Autodesk Inventor part; units mm, degrees
(part 3 of 3)
  spline S531 degree 2 poles (91.9053, 44.1267) (92.1175, 44.1267) (92.457, 44.0701) (92.5051, 44.0362) knots 0 0 0 1 2 2 2
  line L562 (92.5051, 44.0362) -> (92.5051, 43.3289)
  spline S532 degree 2 poles (92.5051, 43.3289) (92.4372, 43.3826) (92.1826, 43.4618) (92.0751, 43.4618) knots 0 0 0 1 2 2 2
  spline S533 degree 2 poles (92.0751, 43.4618) (91.8091, 43.4618) (91.5347, 43.21) (91.5347, 42.9808) knots 0 0 0 1 2 2 2
  spline S534 degree 2 poles (91.5347, 42.9808) (91.5347, 42.7545) (91.8035, 42.5055) (92.0411, 42.5055) knots 0 0 0 1 2 2 2
  spline S535 degree 2 poles (92.0411, 42.5055) (92.2929, 42.5055) (92.5051, 42.6244) knots 0 0 0 1 1 1
  line L563 (92.5051, 42.6244) -> (92.5051, 41.9566)
  spline S536 degree 2 poles (93.6482, 42.7262) (93.6708, 42.5847) (93.9481, 42.4263) (94.1744, 42.4263) knots 0 0 0 1 2 2 2
  spline S537 degree 2 poles (94.1744, 42.4263) (94.4913, 42.4263) (94.7742, 42.548) knots 0 0 0 1 1 1
  line L564 (94.7742, 42.548) -> (94.7742, 41.9736)
  spline S538 degree 2 poles (94.7742, 41.9736) (94.446, 41.8406) (93.9735, 41.8406) knots 0 0 0 1 1 1
  spline S539 degree 2 poles (93.9735, 41.8406) (93.4048, 41.8406) (92.7711, 42.4235) (92.7711, 42.9356) knots 0 0 0 1 2 2 2
  spline S540 degree 2 poles (92.7711, 42.9356) (92.7711, 43.2864) (93.0484, 43.8212) (93.5944, 44.1267) (93.9254, 44.1267) knots 0 0 0 1 2 3 3 3
  spline S541 degree 2 poles (93.9254, 44.1267) (94.2621, 44.1267) (94.7431, 43.8636) (94.9921, 43.3854) (94.9921, 43.0657) knots 0 0 0 1 2 3 3 3
  line L565 (94.9921, 43.0657) -> (94.9921, 42.7262)
  line L566 (94.9921, 42.7262) -> (93.6482, 42.7262)
  spline S542 degree 2 poles (94.1914, 43.2015) (94.1914, 43.5778) (93.9226, 43.5778) knots 0 0 0 1 1 1
  spline S543 degree 2 poles (93.9226, 43.5778) (93.8094, 43.5778) (93.6567, 43.3713) (93.6425, 43.2015) knots 0 0 0 1 2 2 2
  line L567 (93.6425, 43.2015) -> (94.1914, 43.2015)
  line L568 (96.718, 41.8944) -> (96.718, 43.0827)
  spline S544 degree 2 poles (96.718, 43.0827) (96.718, 43.2864) (96.5963, 43.4618) (96.4605, 43.4618) knots 0 0 0 1 2 2 2
  spline S545 degree 2 poles (96.4605, 43.4618) (96.3445, 43.4618) (96.2115, 43.2779) (96.2115, 43.1365) knots 0 0 0 1 2 2 2
  line L569 (96.2115, 43.1365) -> (96.2115, 41.8944)
  line L570 (96.2115, 41.8944) -> (95.3061, 41.8944)
  line L571 (95.3061, 41.8944) -> (95.3061, 44.073)
  line L572 (95.3061, 44.073) -> (96.2115, 44.073)
  line L573 (96.2115, 44.073) -> (96.2115, 43.7334)
  line L574 (96.2115, 43.7334) -> (96.22, 43.7334)
  spline S546 degree 2 poles (96.22, 43.7334) (96.3275, 43.9202) (96.6953, 44.1267) (96.9104, 44.1267) knots 0 0 0 1 2 2 2
  spline S547 degree 2 poles (96.9104, 44.1267) (97.6234, 44.1267) (97.6234, 43.2242) knots 0 0 0 1 1 1
  line L575 (97.6234, 43.2242) -> (97.6234, 41.8944)
  line L576 (97.6234, 41.8944) -> (96.718, 41.8944)
  line L577 (99.0578, 42.5225) -> (99.9547, 42.5225)
  line L578 (99.9547, 42.5225) -> (99.9547, 41.8944)
  line L579 (99.9547, 41.8944) -> (97.8695, 41.8944)
  line L580 (97.8695, 41.8944) -> (97.8695, 42.3131)
  line L581 (97.8695, 42.3131) -> (98.8484, 43.4449)
  line L582 (98.8484, 43.4449) -> (97.96, 43.4449)
  line L583 (97.96, 43.4449) -> (97.96, 44.073)
  line L584 (97.96, 44.073) -> (99.9349, 44.073)
  line L585 (99.9349, 44.073) -> (99.9349, 43.558)
  line L586 (99.9349, 43.558) -> (99.0578, 42.5225)
  spline S548 degree 2 poles (102.6737, 43.0233) (102.6737, 42.4716) (102.0088, 41.8406) (101.4118, 41.8406) knots 0 0 0 1 2 2 2
  spline S549 degree 2 poles (101.4118, 41.8406) (100.8177, 41.8406) (100.1556, 42.4546) (100.1556, 42.9978) knots 0 0 0 1 2 2 2
  spline S550 degree 2 poles (100.1556, 42.9978) (100.1556, 43.343) (100.4668, 43.8551) (101.0412, 44.1267) (101.4146, 44.1267) knots 0 0 0 1 2 3 3 3
  spline S551 degree 2 poles (101.4146, 44.1267) (101.8023, 44.1267) (102.3709, 43.841) (102.6737, 43.3345) (102.6737, 43.0233) knots 0 0 0 1 2 3 3 3
  spline S552 degree 2 poles (101.7542, 43.0176) (101.7542, 43.4618) (101.4146, 43.4618) knots 0 0 0 1 1 1
  spline S553 degree 2 poles (101.4146, 43.4618) (101.0751, 43.4618) (101.0751, 42.9978) knots 0 0 0 1 1 1
  spline S554 degree 2 poles (101.0751, 42.9978) (101.0751, 42.5055) (101.4203, 42.5055) knots 0 0 0 1 1 1
  spline S555 degree 2 poles (101.4203, 42.5055) (101.7542, 42.5055) (101.7542, 43.0176) knots 0 0 0 1 1 1
  line L587 (105.2257, 44.2257) -> (105.2257, 43.6769)
  line L588 (105.2257, 43.6769) -> (106.1311, 43.6769)
  line L589 (106.1311, 43.6769) -> (106.1311, 42.9582)
  line L590 (106.1311, 42.9582) -> (105.2257, 42.9582)
  line L591 (105.2257, 42.9582) -> (105.2257, 41.8944)
  line L592 (105.2257, 41.8944) -> (104.3062, 41.8944)
  line L593 (104.3062, 41.8944) -> (104.3062, 44.9444)
  line L594 (104.3062, 44.9444) -> (106.2188, 44.9444)
  line L595 (106.2188, 44.9444) -> (106.2188, 44.2257)
  line L596 (106.2188, 44.2257) -> (105.2257, 44.2257)
  line L597 (107.7891, 41.8944) -> (107.7891, 42.2254)
  line L598 (107.7891, 42.2254) -> (107.7806, 42.2254)
  spline S556 degree 2 poles (107.7806, 42.2254) (107.5627, 41.8406) (107.1157, 41.8406) knots 0 0 0 1 1 1
  spline S557 degree 2 poles (107.1157, 41.8406) (106.8073, 41.8406) (106.4593, 42.2056) (106.4593, 42.514) knots 0 0 0 1 2 2 2
  spline S558 degree 2 poles (106.4593, 42.514) (106.4593, 43.1563) (107.2487, 43.2581) knots 0 0 0 1 1 1
  line L599 (107.2487, 43.2581) -> (107.7891, 43.3289)
  spline S559 degree 2 poles (107.7891, 43.3289) (107.7891, 43.4364) (107.5967, 43.5722) (107.4354, 43.5722) knots 0 0 0 1 2 2 2
  spline S560 degree 2 poles (107.4354, 43.5722) (107.0704, 43.5722) (106.663, 43.3628) knots 0 0 0 1 1 1
  line L600 (106.663, 43.3628) -> (106.663, 43.9513)
  spline S561 degree 2 poles (106.663, 43.9513) (106.8384, 44.0277) (107.3732, 44.1267) (107.5627, 44.1267) knots 0 0 0 1 2 2 2
  spline S562 degree 2 poles (107.5627, 44.1267) (108.1173, 44.1267) (108.6181, 43.6514) (108.6181, 43.0968) knots 0 0 0 1 2 2 2
  line L601 (108.6181, 43.0968) -> (108.6181, 41.8944)
  line L602 (108.6181, 41.8944) -> (107.7891, 41.8944)
  spline S563 degree 2 poles (107.2515, 42.6357) (107.2515, 42.548) (107.3647, 42.432) (107.4694, 42.432) knots 0 0 0 1 2 2 2
  spline S564 degree 2 poles (107.4694, 42.432) (107.6108, 42.432) (107.7891, 42.6442) (107.7891, 42.8111) knots 0 0 0 1 2 2 2
  line L603 (107.7891, 42.8111) -> (107.7891, 42.8931)
  line L604 (107.7891, 42.8931) -> (107.4807, 42.8507)
  spline S565 degree 2 poles (107.4807, 42.8507) (107.2515, 42.8111) (107.2515, 42.6357) knots 0 0 0 1 1 1
  spline S566 degree 2 poles (111.4813, 43.0488) (111.4813, 42.6923) (111.2465, 42.1405) (110.8108, 41.8406) (110.5363, 41.8406) knots 0 0 0 1 2 3 3 3
  spline S567 degree 2 poles (110.5363, 41.8406) (110.327, 41.8406) (110.0271, 41.9962) (109.9394, 42.1207) knots 0 0 0 1 2 2 2
  line L605 (109.9394, 42.1207) -> (109.9309, 42.1207)
  line L606 (109.9309, 42.1207) -> (109.9309, 41.8944)
  line L607 (109.9309, 41.8944) -> (109.0255, 41.8944)
  line L608 (109.0255, 41.8944) -> (109.0255, 45.1198)
  line L609 (109.0255, 45.1198) -> (109.9309, 45.1198)
  line L610 (109.9309, 45.1198) -> (109.9309, 43.7787)
  line L611 (109.9309, 43.7787) -> (109.9394, 43.7787)
  spline S568 degree 2 poles (109.9394, 43.7787) (110.0469, 43.94) (110.409, 44.1267) (110.6297, 44.1267) knots 0 0 0 1 2 2 2
  spline S569 degree 2 poles (110.6297, 44.1267) (111.04, 44.1267) (111.4813, 43.5778) (111.4813, 43.0488) knots 0 0 0 1 2 2 2
  spline S570 degree 2 poles (110.5618, 43.0233) (110.5618, 43.2411) (110.3949, 43.4618) (110.2364, 43.4618) knots 0 0 0 1 2 2 2
  spline S571 degree 2 poles (110.2364, 43.4618) (110.0978, 43.4618) (109.9139, 43.2298) (109.9139, 43.0459) knots 0 0 0 1 2 2 2
  line L612 (109.9139, 43.0459) -> (109.9139, 42.9129)
  spline S572 degree 2 poles (109.9139, 42.9129) (109.9139, 42.7262) (110.0808, 42.5055) (110.2195, 42.5055) knots 0 0 0 1 2 2 2
  spline S573 degree 2 poles (110.2195, 42.5055) (110.3836, 42.5055) (110.5618, 42.7743) (110.5618, 43.0233) knots 0 0 0 1 2 2 2
  line L613 (111.8237, 41.8944) -> (111.8237, 44.073)
  line L614 (111.8237, 44.073) -> (112.7291, 44.073)
  line L615 (112.7291, 44.073) -> (112.7291, 41.8944)
  line L616 (112.7291, 41.8944) -> (111.8237, 41.8944)
  spline S574 degree 2 poles (112.7828, 44.6615) (112.7828, 44.4691) (112.5027, 44.2314) (112.2764, 44.2314) knots 0 0 0 1 2 2 2
  spline S575 degree 2 poles (112.2764, 44.2314) (112.0557, 44.2314) (111.7728, 44.4776) (111.7728, 44.6615) knots 0 0 0 1 2 2 2
  spline S576 degree 2 poles (111.7728, 44.6615) (111.7728, 44.8482) (112.0472, 45.0802) (112.2764, 45.0802) knots 0 0 0 1 2 2 2
  spline S577 degree 2 poles (112.2764, 45.0802) (112.5027, 45.0802) (112.7828, 44.8482) (112.7828, 44.6615) knots 0 0 0 1 2 2 2
  spline S578 degree 2 poles (115.5867, 43.0233) (115.5867, 42.4716) (114.9218, 41.8406) (114.3248, 41.8406) knots 0 0 0 1 2 2 2
  spline S579 degree 2 poles (114.3248, 41.8406) (113.7306, 41.8406) (113.0686, 42.4546) (113.0686, 42.9978) knots 0 0 0 1 2 2 2
  spline S580 degree 2 poles (113.0686, 42.9978) (113.0686, 43.343) (113.3798, 43.8551) (113.9542, 44.1267) (114.3276, 44.1267) knots 0 0 0 1 2 3 3 3
  spline S581 degree 2 poles (114.3276, 44.1267) (114.7152, 44.1267) (115.2839, 43.841) (115.5867, 43.3345) (115.5867, 43.0233) knots 0 0 0 1 2 3 3 3
  spline S582 degree 2 poles (114.6671, 43.0176) (114.6671, 43.4618) (114.3276, 43.4618) knots 0 0 0 1 1 1
  spline S583 degree 2 poles (114.3276, 43.4618) (113.9881, 43.4618) (113.9881, 42.9978) knots 0 0 0 1 1 1
  spline S584 degree 2 poles (113.9881, 42.9978) (113.9881, 42.5055) (114.3333, 42.5055) knots 0 0 0 1 1 1
  spline S585 degree 2 poles (114.3333, 42.5055) (114.6671, 42.5055) (114.6671, 43.0176) knots 0 0 0 1 1 1
  spline S586 degree 2 poles (69.93, 36.9961) (69.93, 36.832) (69.7603, 36.5406) (69.4689, 36.3736) (69.3076, 36.3736) knots 0 0 0 1 2 3 3 3
  spline S587 degree 2 poles (69.3076, 36.3736) (69.0558, 36.3736) (68.6936, 36.7358) (68.6936, 36.9961) knots 0 0 0 1 2 2 2
  spline S588 degree 2 poles (68.6936, 36.9961) (68.6936, 37.2479) (69.0501, 37.61) (69.3076, 37.61) knots 0 0 0 1 2 2 2
  spline S589 degree 2 poles (69.3076, 37.61) (69.5707, 37.61) (69.93, 37.2422) (69.93, 36.9961) knots 0 0 0 1 2 2 2
  line L617 (80.5994, 35.9577) -> (80.5994, 37.6299)
  spline S590 degree 2 poles (80.5994, 37.6299) (80.5994, 37.8647) (80.6135, 38.1476) knots 0 0 0 1 1 1
  line L618 (80.6135, 38.1476) -> (80.622, 38.2891)
  line L619 (80.622, 38.2891) -> (80.5965, 38.2891)
  spline S591 degree 2 poles (80.5965, 38.2891) (80.5258, 37.9298) (80.4919, 37.7911) knots 0 0 0 1 1 1
  line L620 (80.4919, 37.7911) -> (80.042, 35.9577)
  line L621 (80.042, 35.9577) -> (79.1791, 35.9577)
  line L622 (79.1791, 35.9577) -> (78.7094, 37.7713)
  spline S592 degree 2 poles (78.7094, 37.7713) (78.6896, 37.8392) (78.6075, 38.2891) knots 0 0 0 1 1 1
  line L623 (78.6075, 38.2891) -> (78.5821, 38.2891)
  spline S593 degree 2 poles (78.5821, 38.2891) (78.6132, 37.5733) (78.6132, 37.395) knots 0 0 0 1 1 1
  line L624 (78.6132, 37.395) -> (78.6132, 35.9577)
  line L625 (78.6132, 35.9577) -> (77.8068, 35.9577)
  line L626 (77.8068, 35.9577) -> (77.8068, 39.0077)
  line L627 (77.8068, 39.0077) -> (79.1819, 39.0077)
  line L628 (79.1819, 39.0077) -> (79.6006, 37.3526)
  spline S594 degree 2 poles (79.6006, 37.3526) (79.6176, 37.3017) (79.6657, 36.9876) (79.6714, 36.9027) knots 0 0 0 1 2 2 2
  line L629 (79.6714, 36.9027) -> (79.6855, 36.9027)
  spline S595 degree 2 poles (79.6855, 36.9027) (79.7081, 37.0951) (79.7591, 37.3611) knots 0 0 0 1 1 1
  line L630 (79.7591, 37.3611) -> (80.1495, 39.0077)
  line L631 (80.1495, 39.0077) -> (81.5048, 39.0077)
  line L632 (81.5048, 39.0077) -> (81.5048, 35.9577)
  line L633 (81.5048, 35.9577) -> (80.5994, 35.9577)
  spline S596 degree 2 poles (82.8062, 36.7895) (82.8289, 36.6481) (83.1061, 36.4896) (83.3325, 36.4896) knots 0 0 0 1 2 2 2
  spline S597 degree 2 poles (83.3325, 36.4896) (83.6494, 36.4896) (83.9323, 36.6113) knots 0 0 0 1 1 1
  line L634 (83.9323, 36.6113) -> (83.9323, 36.0369)
  spline S598 degree 2 poles (83.9323, 36.0369) (83.6041, 35.904) (83.1316, 35.904) knots 0 0 0 1 1 1
  spline S599 degree 2 poles (83.1316, 35.904) (82.5629, 35.904) (81.9292, 36.4868) (81.9292, 36.9989) knots 0 0 0 1 2 2 2
  spline S600 degree 2 poles (81.9292, 36.9989) (81.9292, 37.3497) (82.2064, 37.8845) (82.7525, 38.1901) (83.0835, 38.1901) knots 0 0 0 1 2 3 3 3
  spline S601 degree 2 poles (83.0835, 38.1901) (83.4202, 38.1901) (83.9012, 37.9269) (84.1502, 37.4488) (84.1502, 37.1291) knots 0 0 0 1 2 3 3 3
  line L635 (84.1502, 37.1291) -> (84.1502, 36.7895)
  line L636 (84.1502, 36.7895) -> (82.8062, 36.7895)
  spline S602 degree 2 poles (83.3495, 37.2649) (83.3495, 37.6412) (83.0807, 37.6412) knots 0 0 0 1 1 1
  spline S603 degree 2 poles (83.0807, 37.6412) (82.9675, 37.6412) (82.8147, 37.4346) (82.8006, 37.2649) knots 0 0 0 1 2 2 2
  line L637 (82.8006, 37.2649) -> (83.3495, 37.2649)
  line L638 (85.876, 35.9577) -> (85.876, 37.146)
  spline S604 degree 2 poles (85.876, 37.146) (85.876, 37.3497) (85.7544, 37.5252) (85.6186, 37.5252) knots 0 0 0 1 2 2 2
  spline S605 degree 2 poles (85.6186, 37.5252) (85.5026, 37.5252) (85.3696, 37.3413) (85.3696, 37.1998) knots 0 0 0 1 2 2 2
  line L639 (85.3696, 37.1998) -> (85.3696, 35.9577)
  line L640 (85.3696, 35.9577) -> (84.4642, 35.9577)
  line L641 (84.4642, 35.9577) -> (84.4642, 38.1363)
  line L642 (84.4642, 38.1363) -> (85.3696, 38.1363)
  line L643 (85.3696, 38.1363) -> (85.3696, 37.7968)
  line L644 (85.3696, 37.7968) -> (85.3781, 37.7968)
  spline S606 degree 2 poles (85.3781, 37.7968) (85.4856, 37.9835) (85.8534, 38.1901) (86.0684, 38.1901) knots 0 0 0 1 2 2 2
  spline S607 degree 2 poles (86.0684, 38.1901) (86.7814, 38.1901) (86.7814, 37.2875) knots 0 0 0 1 1 1
  line L645 (86.7814, 37.2875) -> (86.7814, 35.9577)
  line L646 (86.7814, 35.9577) -> (85.876, 35.9577)
  line L647 (87.1917, 35.9577) -> (87.1917, 38.1363)
  line L648 (87.1917, 38.1363) -> (88.0971, 38.1363)
  line L649 (88.0971, 38.1363) -> (88.0971, 35.9577)
  line L650 (88.0971, 35.9577) -> (87.1917, 35.9577)
  spline S608 degree 2 poles (88.1508, 38.7248) (88.1508, 38.5324) (87.8707, 38.2947) (87.6444, 38.2947) knots 0 0 0 1 2 2 2
  spline S609 degree 2 poles (87.6444, 38.2947) (87.4237, 38.2947) (87.1407, 38.5409) (87.1407, 38.7248) knots 0 0 0 1 2 2 2
  spline S610 degree 2 poles (87.1407, 38.7248) (87.1407, 38.9115) (87.4152, 39.1435) (87.6444, 39.1435) knots 0 0 0 1 2 2 2
  spline S611 degree 2 poles (87.6444, 39.1435) (87.8707, 39.1435) (88.1508, 38.9115) (88.1508, 38.7248) knots 0 0 0 1 2 2 2
  spline S612 degree 2 poles (90.3266, 36.02) (90.2388, 35.969) (89.8654, 35.904) (89.6221, 35.904) knots 0 0 0 1 2 2 2
  spline S613 degree 2 poles (89.6221, 35.904) (89.2769, 35.904) (88.7337, 36.1841) (88.4366, 36.6849) (88.4366, 36.9989) knots 0 0 0 1 2 3 3 3
  spline S614 degree 2 poles (88.4366, 36.9989) (88.4366, 37.3724) (88.7535, 37.9071) (89.3391, 38.1901) (89.7267, 38.1901) knots 0 0 0 1 2 3 3 3
  spline S615 degree 2 poles (89.7267, 38.1901) (89.9389, 38.1901) (90.2785, 38.1335) (90.3266, 38.0995) knots 0 0 0 1 2 2 2
  line L651 (90.3266, 38.0995) -> (90.3266, 37.3922)
  spline S616 degree 2 poles (90.3266, 37.3922) (90.2587, 37.4459) (90.004, 37.5252) (89.8965, 37.5252) knots 0 0 0 1 2 2 2
  spline S617 degree 2 poles (89.8965, 37.5252) (89.6305, 37.5252) (89.3561, 37.2734) (89.3561, 37.0442) knots 0 0 0 1 2 2 2
  spline S618 degree 2 poles (89.3561, 37.0442) (89.3561, 36.8178) (89.6249, 36.5689) (89.8625, 36.5689) knots 0 0 0 1 2 2 2
  spline S619 degree 2 poles (89.8625, 36.5689) (90.1144, 36.5689) (90.3266, 36.6877) knots 0 0 0 1 1 1
  line L652 (90.3266, 36.6877) -> (90.3266, 36.02)
  line L653 (92.092, 35.9577) -> (92.092, 37.1998)
  spline S620 degree 2 poles (92.092, 37.1998) (92.092, 37.5252) (91.8431, 37.5252) knots 0 0 0 1 1 1
  spline S621 degree 2 poles (91.8431, 37.5252) (91.7214, 37.5252) (91.5941, 37.3413) (91.5941, 37.1941) knots 0 0 0 1 2 2 2
  line L654 (91.5941, 37.1941) -> (91.5941, 35.9577)
  line L655 (91.5941, 35.9577) -> (90.6887, 35.9577)
  line L656 (90.6887, 35.9577) -> (90.6887, 39.1831)
  line L657 (90.6887, 39.1831) -> (91.5941, 39.1831)
  line L658 (91.5941, 39.1831) -> (91.5941, 37.842)
  line L659 (91.5941, 37.842) -> (91.6026, 37.842)
  spline S622 degree 2 poles (91.6026, 37.842) (91.7186, 38.009) (92.0553, 38.1901) (92.2448, 38.1901) knots 0 0 0 1 2 2 2
  spline S623 degree 2 poles (92.2448, 38.1901) (92.5985, 38.1901) (92.9691, 37.7374) (92.9691, 37.296) knots 0 0 0 1 2 2 2
  line L660 (92.9691, 37.296) -> (92.9691, 35.9577)
  line L661 (92.9691, 35.9577) -> (92.092, 35.9577)
  spline S624 degree 2 poles (94.1574, 36.7895) (94.1801, 36.6481) (94.4574, 36.4896) (94.6837, 36.4896) knots 0 0 0 1 2 2 2
  spline S625 degree 2 poles (94.6837, 36.4896) (95.0006, 36.4896) (95.2835, 36.6113) knots 0 0 0 1 1 1
  line L662 (95.2835, 36.6113) -> (95.2835, 36.0369)
  spline S626 degree 2 poles (95.2835, 36.0369) (94.9553, 35.904) (94.4828, 35.904) knots 0 0 0 1 1 1
  spline S627 degree 2 poles (94.4828, 35.904) (93.9141, 35.904) (93.2804, 36.4868) (93.2804, 36.9989) knots 0 0 0 1 2 2 2
  spline S628 degree 2 poles (93.2804, 36.9989) (93.2804, 37.3497) (93.5576, 37.8845) (94.1037, 38.1901) (94.4347, 38.1901) knots 0 0 0 1 2 3 3 3
  spline S629 degree 2 poles (94.4347, 38.1901) (94.7714, 38.1901) (95.2524, 37.9269) (95.5014, 37.4488) (95.5014, 37.1291) knots 0 0 0 1 2 3 3 3
  line L663 (95.5014, 37.1291) -> (95.5014, 36.7895)
  line L664 (95.5014, 36.7895) -> (94.1574, 36.7895)
  spline S630 degree 2 poles (94.7007, 37.2649) (94.7007, 37.6412) (94.4319, 37.6412) knots 0 0 0 1 1 1
  spline S631 degree 2 poles (94.4319, 37.6412) (94.3187, 37.6412) (94.1659, 37.4346) (94.1518, 37.2649) knots 0 0 0 1 2 2 2
  line L665 (94.1518, 37.2649) -> (94.7007, 37.2649)
  line L666 (95.8154, 35.9577) -> (95.8154, 39.1831)
  line L667 (95.8154, 39.1831) -> (96.7208, 39.1831)
  line L668 (96.7208, 39.1831) -> (96.7208, 35.9577)
  line L669 (96.7208, 35.9577) -> (95.8154, 35.9577)
  line L670 (97.1565, 35.9577) -> (97.1565, 39.1831)
  line L671 (97.1565, 39.1831) -> (98.0619, 39.1831)
  line L672 (98.0619, 39.1831) -> (98.0619, 35.9577)
  line L673 (98.0619, 35.9577) -> (97.1565, 35.9577)
  line L674 (98.4976, 35.9577) -> (98.4976, 38.1363)
  line L675 (98.4976, 38.1363) -> (99.403, 38.1363)
  line L676 (99.403, 38.1363) -> (99.403, 35.9577)
  line L677 (99.403, 35.9577) -> (98.4976, 35.9577)
  spline S632 degree 2 poles (99.4568, 38.7248) (99.4568, 38.5324) (99.1766, 38.2947) (98.9503, 38.2947) knots 0 0 0 1 2 2 2
  spline S633 degree 2 poles (98.9503, 38.2947) (98.7296, 38.2947) (98.4467, 38.5409) (98.4467, 38.7248) knots 0 0 0 1 2 2 2
  spline S634 degree 2 poles (98.4467, 38.7248) (98.4467, 38.9115) (98.7211, 39.1435) (98.9503, 39.1435) knots 0 0 0 1 2 2 2
  spline S635 degree 2 poles (98.9503, 39.1435) (99.1766, 39.1435) (99.4568, 38.9115) (99.4568, 38.7248) knots 0 0 0 1 2 2 2
  line L678 (103.0443, 35.9577) -> (102.9113, 36.5179)
  line L679 (102.9113, 36.5179) -> (102.0003, 36.5179)
  line L680 (102.0003, 36.5179) -> (101.856, 35.9577)
  line L681 (101.856, 35.9577) -> (100.8629, 35.9577)
  line L682 (100.8629, 35.9577) -> (101.9126, 39.0077)
  line L683 (101.9126, 39.0077) -> (103.0528, 39.0077)
  line L684 (103.0528, 39.0077) -> (104.0431, 35.9577)
  line L685 (104.0431, 35.9577) -> (103.0443, 35.9577)
  line L686 (102.4671, 38.3428) -> (102.4473, 38.3428)
  spline S636 degree 2 poles (102.4473, 38.3428) (102.4417, 38.2919) (102.3907, 38.0571) (102.1587, 37.1715) knots 0 0 0 1 2 2 2
  line L687 (102.1587, 37.1715) -> (102.7416, 37.1715)
  line L688 (102.7416, 37.1715) -> (102.5294, 38.0005)
  spline S637 degree 2 poles (102.5294, 38.0005) (102.4841, 38.1844) (102.4671, 38.3428) knots 0 0 0 1 1 1
  line L689 (104.3175, 35.9577) -> (104.3175, 39.1831)
  line L690 (104.3175, 39.1831) -> (105.2229, 39.1831)
  line L691 (105.2229, 39.1831) -> (105.2229, 35.9577)
  line L692 (105.2229, 35.9577) -> (104.3175, 35.9577)
  spline S638 degree 2 poles (108.1145, 37.1121) (108.1145, 36.7556) (107.8796, 36.2039) (107.4439, 35.904) (107.1695, 35.904) knots 0 0 0 1 2 3 3 3
  spline S639 degree 2 poles (107.1695, 35.904) (106.9601, 35.904) (106.6602, 36.0596) (106.5725, 36.1841) knots 0 0 0 1 2 2 2
  line L693 (106.5725, 36.1841) -> (106.564, 36.1841)
  line L694 (106.564, 36.1841) -> (106.564, 35.9577)
  line L695 (106.564, 35.9577) -> (105.6586, 35.9577)
  line L696 (105.6586, 35.9577) -> (105.6586, 39.1831)
  line L697 (105.6586, 39.1831) -> (106.564, 39.1831)
  line L698 (106.564, 39.1831) -> (106.564, 37.842)
  line L699 (106.564, 37.842) -> (106.5725, 37.842)
  spline S640 degree 2 poles (106.5725, 37.842) (106.68, 38.0033) (107.0421, 38.1901) (107.2628, 38.1901) knots 0 0 0 1 2 2 2
  spline S641 degree 2 poles (107.2628, 38.1901) (107.6731, 38.1901) (108.1145, 37.6412) (108.1145, 37.1121) knots 0 0 0 1 2 2 2
  spline S642 degree 2 poles (107.1949, 37.0866) (107.1949, 37.3045) (107.028, 37.5252) (106.8696, 37.5252) knots 0 0 0 1 2 2 2
  spline S643 degree 2 poles (106.8696, 37.5252) (106.7309, 37.5252) (106.547, 37.2932) (106.547, 37.1093) knots 0 0 0 1 2 2 2
  line L700 (106.547, 37.1093) -> (106.547, 36.9763)
  spline S644 degree 2 poles (106.547, 36.9763) (106.547, 36.7895) (106.7139, 36.5689) (106.8526, 36.5689) knots 0 0 0 1 2 2 2
  spline S645 degree 2 poles (106.8526, 36.5689) (107.0167, 36.5689) (107.1949, 36.8376) (107.1949, 37.0866) knots 0 0 0 1 2 2 2
  spline S646 degree 2 poles (109.2377, 36.7895) (109.2603, 36.6481) (109.5376, 36.4896) (109.7639, 36.4896) knots 0 0 0 1 2 2 2
  spline S647 degree 2 poles (109.7639, 36.4896) (110.0808, 36.4896) (110.3638, 36.6113) knots 0 0 0 1 1 1
  line L701 (110.3638, 36.6113) -> (110.3638, 36.0369)
  spline S648 degree 2 poles (110.3638, 36.0369) (110.0356, 35.904) (109.5631, 35.904) knots 0 0 0 1 1 1
  spline S649 degree 2 poles (109.5631, 35.904) (108.9944, 35.904) (108.3606, 36.4868) (108.3606, 36.9989) knots 0 0 0 1 2 2 2
  spline S650 degree 2 poles (108.3606, 36.9989) (108.3606, 37.3497) (108.6379, 37.8845) (109.1839, 38.1901) (109.515, 38.1901) knots 0 0 0 1 2 3 3 3
  spline S651 degree 2 poles (109.515, 38.1901) (109.8516, 38.1901) (110.3326, 37.9269) (110.5816, 37.4488) (110.5816, 37.1291) knots 0 0 0 1 2 3 3 3
  line L702 (110.5816, 37.1291) -> (110.5816, 36.7895)
  line L703 (110.5816, 36.7895) -> (109.2377, 36.7895)
  spline S652 degree 2 poles (109.7809, 37.2649) (109.7809, 37.6412) (109.5121, 37.6412) knots 0 0 0 1 1 1
  spline S653 degree 2 poles (109.5121, 37.6412) (109.399, 37.6412) (109.2462, 37.4346) (109.232, 37.2649) knots 0 0 0 1 2 2 2
  line L704 (109.232, 37.2649) -> (109.7809, 37.2649)
  spline S654 degree 2 poles (112.5338, 37.3611) (112.4829, 37.3837) (112.3075, 37.4205) (112.2509, 37.4205) knots 0 0 0 1 2 2 2
  spline S655 degree 2 poles (112.2509, 37.4205) (111.801, 37.4205) (111.801, 36.9027) knots 0 0 0 1 1 1
  line L705 (111.801, 36.9027) -> (111.801, 35.9577)
  line L706 (111.801, 35.9577) -> (110.8957, 35.9577)
  line L707 (110.8957, 35.9577) -> (110.8957, 38.1363)
  line L708 (110.8957, 38.1363) -> (111.801, 38.1363)
  line L709 (111.801, 38.1363) -> (111.801, 37.7543)
  line L710 (111.801, 37.7543) -> (111.8095, 37.7543)
  spline S656 degree 2 poles (111.8095, 37.7543) (111.8916, 37.9609) (112.2, 38.1759) (112.4037, 38.1759) knots 0 0 0 1 2 2 2
  spline S657 degree 2 poles (112.4037, 38.1759) (112.4773, 38.1759) (112.5338, 38.1504) knots 0 0 0 1 1 1
  line L711 (112.5338, 38.1504) -> (112.5338, 37.3611)
  spline S658 degree 2 poles (114.3276, 35.986) (114.2654, 35.9577) (113.9853, 35.904) (113.7872, 35.904) knots 0 0 0 1 2 2 2
  spline S659 degree 2 poles (113.7872, 35.904) (113.4081, 35.904) (112.9809, 36.3199) (112.9809, 36.7075) knots 0 0 0 1 2 2 2
  line L712 (112.9809, 36.7075) -> (112.9809, 37.5082)
  line L713 (112.9809, 37.5082) -> (112.6385, 37.5082)
  line L714 (112.6385, 37.5082) -> (112.6385, 38.1363)
  line L715 (112.6385, 38.1363) -> (112.9809, 38.1363)
  line L716 (112.9809, 38.1363) -> (112.9809, 38.5635)
  line L717 (112.9809, 38.5635) -> (113.8749, 38.8097)
  line L718 (113.8749, 38.8097) -> (113.8749, 38.1363)
  line L719 (113.8749, 38.1363) -> (114.3276, 38.1363)
  line L720 (114.3276, 38.1363) -> (114.3276, 37.5082)
  line L721 (114.3276, 37.5082) -> (113.8749, 37.5082)
  line L722 (113.8749, 37.5082) -> (113.8749, 36.8546)
  spline S660 degree 2 poles (113.8749, 36.8546) (113.8749, 36.5689) (114.1013, 36.5689) knots 0 0 0 1 1 1
  spline S661 degree 2 poles (114.1013, 36.5689) (114.2088, 36.5689) (114.3276, 36.6141) knots 0 0 0 1 1 1
  line L723 (114.3276, 36.6141) -> (114.3276, 35.986)
  spline S662 degree 2 poles (117.0324, 37.0866) (117.0324, 36.5349) (116.3676, 35.904) (115.7706, 35.904) knots 0 0 0 1 2 2 2
  spline S663 degree 2 poles (115.7706, 35.904) (115.1764, 35.904) (114.5144, 36.5179) (114.5144, 37.0612) knots 0 0 0 1 2 2 2
  spline S664 degree 2 poles (114.5144, 37.0612) (114.5144, 37.4063) (114.8256, 37.9184) (115.3999, 38.1901) (115.7734, 38.1901) knots 0 0 0 1 2 3 3 3
  spline S665 degree 2 poles (115.7734, 38.1901) (116.161, 38.1901) (116.7297, 37.9043) (117.0324, 37.3978) (117.0324, 37.0866) knots 0 0 0 1 2 3 3 3
  spline S666 degree 2 poles (116.1129, 37.081) (116.1129, 37.5252) (115.7734, 37.5252) knots 0 0 0 1 1 1
  spline S667 degree 2 poles (115.7734, 37.5252) (115.4339, 37.5252) (115.4339, 37.0612) knots 0 0 0 1 1 1
  spline S668 degree 2 poles (115.4339, 37.0612) (115.4339, 36.5689) (115.7791, 36.5689) knots 0 0 0 1 1 1
  spline S669 degree 2 poles (115.7791, 36.5689) (116.1129, 36.5689) (116.1129, 37.081) knots 0 0 0 1 1 1
  spline S670 degree 2 poles (69.93, 31.0594) (69.93, 30.8953) (69.7603, 30.6039) (69.4689, 30.437) (69.3076, 30.437) knots 0 0 0 1 2 3 3 3
  spline S671 degree 2 poles (69.3076, 30.437) (69.0558, 30.437) (68.6936, 30.7991) (68.6936, 31.0594) knots 0 0 0 1 2 2 2
  spline S672 degree 2 poles (68.6936, 31.0594) (68.6936, 31.3112) (69.0501, 31.6734) (69.3076, 31.6734) knots 0 0 0 1 2 2 2
  spline S673 degree 2 poles (69.3076, 31.6734) (69.5707, 31.6734) (69.93, 31.3056) (69.93, 31.0594) knots 0 0 0 1 2 2 2
  line L724 (78.7264, 32.3524) -> (78.7264, 31.8035)
  line L725 (78.7264, 31.8035) -> (79.6318, 31.8035)
  line L726 (79.6318, 31.8035) -> (79.6318, 31.0849)
  line L727 (79.6318, 31.0849) -> (78.7264, 31.0849)
  line L728 (78.7264, 31.0849) -> (78.7264, 30.0211)
  line L729 (78.7264, 30.0211) -> (77.8068, 30.0211)
  line L730 (77.8068, 30.0211) -> (77.8068, 33.0711)
  line L731 (77.8068, 33.0711) -> (79.7195, 33.0711)
  line L732 (79.7195, 33.0711) -> (79.7195, 32.3524)
  line L733 (79.7195, 32.3524) -> (78.7264, 32.3524)
  spline S674 degree 2 poles (80.8625, 30.8529) (80.8851, 30.7114) (81.1624, 30.553) (81.3888, 30.553) knots 0 0 0 1 2 2 2
  spline S675 degree 2 poles (81.3888, 30.553) (81.7056, 30.553) (81.9886, 30.6746) knots 0 0 0 1 1 1
  line L734 (81.9886, 30.6746) -> (81.9886, 30.1003)
  spline S676 degree 2 poles (81.9886, 30.1003) (81.6604, 29.9673) (81.1879, 29.9673) knots 0 0 0 1 1 1
  spline S677 degree 2 poles (81.1879, 29.9673) (80.6192, 29.9673) (79.9854, 30.5501) (79.9854, 31.0622) knots 0 0 0 1 2 2 2
  spline S678 degree 2 poles (79.9854, 31.0622) (79.9854, 31.4131) (80.2627, 31.9478) (80.8087, 32.2534) (81.1398, 32.2534) knots 0 0 0 1 2 3 3 3
  spline S679 degree 2 poles (81.1398, 32.2534) (81.4765, 32.2534) (81.9574, 31.9903) (82.2064, 31.5121) (82.2064, 31.1924) knots 0 0 0 1 2 3 3 3
  line L735 (82.2064, 31.1924) -> (82.2064, 30.8529)
  line L736 (82.2064, 30.8529) -> (80.8625, 30.8529)
  spline S680 degree 2 poles (81.4057, 31.3282) (81.4057, 31.7045) (81.1369, 31.7045) knots 0 0 0 1 1 1
  spline S681 degree 2 poles (81.1369, 31.7045) (81.0238, 31.7045) (80.871, 31.498) (80.8568, 31.3282) knots 0 0 0 1 2 2 2
  line L737 (80.8568, 31.3282) -> (81.4057, 31.3282)
  spline S682 degree 2 poles (84.1587, 31.4244) (84.1077, 31.447) (83.9323, 31.4838) (83.8757, 31.4838) knots 0 0 0 1 2 2 2
  spline S683 degree 2 poles (83.8757, 31.4838) (83.4259, 31.4838) (83.4259, 30.9661) knots 0 0 0 1 1 1
  line L738 (83.4259, 30.9661) -> (83.4259, 30.0211)
  line L739 (83.4259, 30.0211) -> (82.5205, 30.0211)
  line L740 (82.5205, 30.0211) -> (82.5205, 32.1996)
  line L741 (82.5205, 32.1996) -> (83.4259, 32.1996)
  line L742 (83.4259, 32.1996) -> (83.4259, 31.8177)
  line L743 (83.4259, 31.8177) -> (83.4343, 31.8177)
  spline S684 degree 2 poles (83.4343, 31.8177) (83.5164, 32.0242) (83.8248, 32.2392) (84.0285, 32.2392) knots 0 0 0 1 2 2 2
  spline S685 degree 2 poles (84.0285, 32.2392) (84.1021, 32.2392) (84.1587, 32.2138) knots 0 0 0 1 1 1
  line L744 (84.1587, 32.2138) -> (84.1587, 31.4244)
  spline S686 degree 2 poles (86.0571, 31.4244) (86.0062, 31.447) (85.8308, 31.4838) (85.7742, 31.4838) knots 0 0 0 1 2 2 2
  spline S687 degree 2 poles (85.7742, 31.4838) (85.3243, 31.4838) (85.3243, 30.9661) knots 0 0 0 1 1 1
  line L745 (85.3243, 30.9661) -> (85.3243, 30.0211)
  line L746 (85.3243, 30.0211) -> (84.4189, 30.0211)
  line L747 (84.4189, 30.0211) -> (84.4189, 32.1996)
  line L748 (84.4189, 32.1996) -> (85.3243, 32.1996)
  line L749 (85.3243, 32.1996) -> (85.3243, 31.8177)
  line L750 (85.3243, 31.8177) -> (85.3328, 31.8177)
  spline S688 degree 2 poles (85.3328, 31.8177) (85.4149, 32.0242) (85.7233, 32.2392) (85.927, 32.2392) knots 0 0 0 1 2 2 2
  spline S689 degree 2 poles (85.927, 32.2392) (86.0005, 32.2392) (86.0571, 32.2138) knots 0 0 0 1 1 1
  line L751 (86.0571, 32.2138) -> (86.0571, 31.4244)
  spline S690 degree 2 poles (88.7393, 31.15) (88.7393, 30.5982) (88.0744, 29.9673) (87.4774, 29.9673) knots 0 0 0 1 2 2 2
  spline S691 degree 2 poles (87.4774, 29.9673) (86.8833, 29.9673) (86.2212, 30.5813) (86.2212, 31.1245) knots 0 0 0 1 2 2 2
  spline S692 degree 2 poles (86.2212, 31.1245) (86.2212, 31.4697) (86.5324, 31.9818) (87.1068, 32.2534) (87.4803, 32.2534) knots 0 0 0 1 2 3 3 3
  spline S693 degree 2 poles (87.4803, 32.2534) (87.8679, 32.2534) (88.4366, 31.9676) (88.7393, 31.4612) (88.7393, 31.15) knots 0 0 0 1 2 3 3 3
  spline S694 degree 2 poles (87.8198, 31.1443) (87.8198, 31.5885) (87.4803, 31.5885) knots 0 0 0 1 1 1
  spline S695 degree 2 poles (87.4803, 31.5885) (87.1407, 31.5885) (87.1407, 31.1245) knots 0 0 0 1 1 1
  spline S696 degree 2 poles (87.1407, 31.1245) (87.1407, 30.6322) (87.4859, 30.6322) knots 0 0 0 1 1 1
  spline S697 degree 2 poles (87.4859, 30.6322) (87.8198, 30.6322) (87.8198, 31.1443) knots 0 0 0 1 1 1
  line L752 (87.3728, 32.5448) -> (86.6145, 33.2267)
  line L753 (86.6145, 33.2267) -> (87.3756, 33.2267)
  line L754 (87.3756, 33.2267) -> (88.0122, 32.5448)
  line L755 (88.0122, 32.5448) -> (87.3728, 32.5448)
  line L756 (91.2914, 32.3524) -> (91.2914, 31.8035)
  line L757 (91.2914, 31.8035) -> (92.1967, 31.8035)
  line L758 (92.1967, 31.8035) -> (92.1967, 31.0849)
  line L759 (92.1967, 31.0849) -> (91.2914, 31.0849)
  line L760 (91.2914, 31.0849) -> (91.2914, 30.0211)
  line L761 (91.2914, 30.0211) -> (90.3718, 30.0211)
  line L762 (90.3718, 30.0211) -> (90.3718, 33.0711)
  line L763 (90.3718, 33.0711) -> (92.2844, 33.0711)
  line L764 (92.2844, 33.0711) -> (92.2844, 32.3524)
  line L765 (92.2844, 32.3524) -> (91.2914, 32.3524)
  spline S698 degree 2 poles (94.2848, 31.4244) (94.2338, 31.447) (94.0584, 31.4838) (94.0018, 31.4838) knots 0 0 0 1 2 2 2
  spline S699 degree 2 poles (94.0018, 31.4838) (93.552, 31.4838) (93.552, 30.9661) knots 0 0 0 1 1 1
  line L766 (93.552, 30.9661) -> (93.552, 30.0211)
  line L767 (93.552, 30.0211) -> (92.6466, 30.0211)
  line L768 (92.6466, 30.0211) -> (92.6466, 32.1996)
  line L769 (92.6466, 32.1996) -> (93.552, 32.1996)
  line L770 (93.552, 32.1996) -> (93.552, 31.8177)
  line L771 (93.552, 31.8177) -> (93.5605, 31.8177)
  spline S700 degree 2 poles (93.5605, 31.8177) (93.6425, 32.0242) (93.9509, 32.2392) (94.1546, 32.2392) knots 0 0 0 1 2 2 2
  spline S701 degree 2 poles (94.1546, 32.2392) (94.2282, 32.2392) (94.2848, 32.2138) knots 0 0 0 1 1 1
  line L772 (94.2848, 32.2138) -> (94.2848, 31.4244)
  line L773 (95.7532, 30.0211) -> (95.7532, 30.3521)
  line L774 (95.7532, 30.3521) -> (95.7447, 30.3521)
  spline S702 degree 2 poles (95.7447, 30.3521) (95.5268, 29.9673) (95.0798, 29.9673) knots 0 0 0 1 1 1
  spline S703 degree 2 poles (95.0798, 29.9673) (94.7714, 29.9673) (94.4234, 30.3323) (94.4234, 30.6407) knots 0 0 0 1 2 2 2
  spline S704 degree 2 poles (94.4234, 30.6407) (94.4234, 31.2829) (95.2128, 31.3848) knots 0 0 0 1 1 1
  line L775 (95.2128, 31.3848) -> (95.7532, 31.4555)
  spline S705 degree 2 poles (95.7532, 31.4555) (95.7532, 31.563) (95.5608, 31.6988) (95.3995, 31.6988) knots 0 0 0 1 2 2 2
  spline S706 degree 2 poles (95.3995, 31.6988) (95.0345, 31.6988) (94.6271, 31.4895) knots 0 0 0 1 1 1
  line L776 (94.6271, 31.4895) -> (94.6271, 32.078)
  spline S707 degree 2 poles (94.6271, 32.078) (94.8025, 32.1544) (95.3373, 32.2534) (95.5268, 32.2534) knots 0 0 0 1 2 2 2
  spline S708 degree 2 poles (95.5268, 32.2534) (96.0814, 32.2534) (96.5822, 31.7781) (96.5822, 31.2235) knots 0 0 0 1 2 2 2
  line L777 (96.5822, 31.2235) -> (96.5822, 30.0211)
  line L778 (96.5822, 30.0211) -> (95.7532, 30.0211)
  spline S709 degree 2 poles (95.2156, 30.7623) (95.2156, 30.6746) (95.3288, 30.5586) (95.4335, 30.5586) knots 0 0 0 1 2 2 2
  spline S710 degree 2 poles (95.4335, 30.5586) (95.5749, 30.5586) (95.7532, 30.7708) (95.7532, 30.9378) knots 0 0 0 1 2 2 2
  line L779 (95.7532, 30.9378) -> (95.7532, 31.0198)
  line L780 (95.7532, 31.0198) -> (95.4448, 30.9774)
  spline S711 degree 2 poles (95.4448, 30.9774) (95.2156, 30.9378) (95.2156, 30.7623) knots 0 0 0 1 1 1
  line L781 (98.4014, 30.0211) -> (98.4014, 31.2094)
  spline S712 degree 2 poles (98.4014, 31.2094) (98.4014, 31.4131) (98.2798, 31.5885) (98.1439, 31.5885) knots 0 0 0 1 2 2 2
  spline S713 degree 2 poles (98.1439, 31.5885) (98.0279, 31.5885) (97.895, 31.4046) (97.895, 31.2631) knots 0 0 0 1 2 2 2
  line L782 (97.895, 31.2631) -> (97.895, 30.0211)
  line L783 (97.895, 30.0211) -> (96.9896, 30.0211)
  line L784 (96.9896, 30.0211) -> (96.9896, 32.1996)
  line L785 (96.9896, 32.1996) -> (97.895, 32.1996)
  line L786 (97.895, 32.1996) -> (97.895, 31.8601)
  line L787 (97.895, 31.8601) -> (97.9035, 31.8601)
  spline S714 degree 2 poles (97.9035, 31.8601) (98.011, 32.0469) (98.3788, 32.2534) (98.5938, 32.2534) knots 0 0 0 1 2 2 2
  spline S715 degree 2 poles (98.5938, 32.2534) (99.3068, 32.2534) (99.3068, 31.3508) knots 0 0 0 1 1 1
  line L788 (99.3068, 31.3508) -> (99.3068, 30.0211)
  line L789 (99.3068, 30.0211) -> (98.4014, 30.0211)
  spline S716 degree 2 poles (101.5108, 30.0833) (101.4231, 30.0324) (101.0497, 29.9673) (100.8063, 29.9673) knots 0 0 0 1 2 2 2
  spline S717 degree 2 poles (100.8063, 29.9673) (100.4612, 29.9673) (99.9179, 30.2474) (99.6209, 30.7482) (99.6209, 31.0622) knots 0 0 0 1 2 3 3 3
  spline S718 degree 2 poles (99.6209, 31.0622) (99.6209, 31.4357) (99.9377, 31.9705) (100.5234, 32.2534) (100.911, 32.2534) knots 0 0 0 1 2 3 3 3
  spline S719 degree 2 poles (100.911, 32.2534) (101.1232, 32.2534) (101.4627, 32.1968) (101.5108, 32.1629) knots 0 0 0 1 2 2 2
  line L790 (101.5108, 32.1629) -> (101.5108, 31.4555)
  spline S720 degree 2 poles (101.5108, 31.4555) (101.4429, 31.5093) (101.1883, 31.5885) (101.0808, 31.5885) knots 0 0 0 1 2 2 2
  spline S721 degree 2 poles (101.0808, 31.5885) (100.8148, 31.5885) (100.5404, 31.3367) (100.5404, 31.1075) knots 0 0 0 1 2 2 2
  spline S722 degree 2 poles (100.5404, 31.1075) (100.5404, 30.8812) (100.8092, 30.6322) (101.0468, 30.6322) knots 0 0 0 1 2 2 2
  spline S723 degree 2 poles (101.0468, 30.6322) (101.2986, 30.6322) (101.5108, 30.751) knots 0 0 0 1 1 1
  line L791 (101.5108, 30.751) -> (101.5108, 30.0833)
  spline S724 degree 2 poles (102.6539, 30.8529) (102.6765, 30.7114) (102.9538, 30.553) (103.1801, 30.553) knots 0 0 0 1 2 2 2
  spline S725 degree 2 poles (103.1801, 30.553) (103.497, 30.553) (103.7799, 30.6746) knots 0 0 0 1 1 1
  line L792 (103.7799, 30.6746) -> (103.7799, 30.1003)
  spline S726 degree 2 poles (103.7799, 30.1003) (103.4517, 29.9673) (102.9792, 29.9673) knots 0 0 0 1 1 1
  spline S727 degree 2 poles (102.9792, 29.9673) (102.4106, 29.9673) (101.7768, 30.5501) (101.7768, 31.0622) knots 0 0 0 1 2 2 2
  spline S728 degree 2 poles (101.7768, 31.0622) (101.7768, 31.4131) (102.0541, 31.9478) (102.6001, 32.2534) (102.9311, 32.2534) knots 0 0 0 1 2 3 3 3
  spline S729 degree 2 poles (102.9311, 32.2534) (103.2678, 32.2534) (103.7488, 31.9903) (103.9978, 31.5121) (103.9978, 31.1924) knots 0 0 0 1 2 3 3 3
  line L793 (103.9978, 31.1924) -> (103.9978, 30.8529)
  line L794 (103.9978, 30.8529) -> (102.6539, 30.8529)
  spline S730 degree 2 poles (103.1971, 31.3282) (103.1971, 31.7045) (102.9283, 31.7045) knots 0 0 0 1 1 1
  spline S731 degree 2 poles (102.9283, 31.7045) (102.8151, 31.7045) (102.6624, 31.498) (102.6482, 31.3282) knots 0 0 0 1 2 2 2
  line L795 (102.6482, 31.3282) -> (103.1971, 31.3282)
  spline S732 degree 2 poles (106.083, 30.7454) (106.083, 30.3747) (105.5171, 29.9673) (105.0135, 29.9673) knots 0 0 0 1 2 2 2
  spline S733 degree 2 poles (105.0135, 29.9673) (104.8664, 29.9673) (104.4335, 30.0267) (104.2977, 30.0692) knots 0 0 0 1 2 2 2
  line L796 (104.2977, 30.0692) -> (104.2977, 30.7058)
  spline S734 degree 2 poles (104.2977, 30.7058) (104.6995, 30.5275) (104.9711, 30.5275) knots 0 0 0 1 1 1
  spline S735 degree 2 poles (104.9711, 30.5275) (105.237, 30.5275) (105.237, 30.6661) knots 0 0 0 1 1 1
  spline S736 degree 2 poles (105.237, 30.6661) (105.237, 30.7227) (105.1125, 30.7991) (104.8523, 30.884) knots 0 0 0 1 2 2 2
  spline S737 degree 2 poles (104.8523, 30.884) (104.5608, 30.9774) (104.2977, 31.2801) (104.2977, 31.5206) knots 0 0 0 1 2 2 2
  spline S738 degree 2 poles (104.2977, 31.5206) (104.2977, 31.8601) (104.8381, 32.2534) (105.3247, 32.2534) knots 0 0 0 1 2 2 2
  spline S739 degree 2 poles (105.3247, 32.2534) (105.6105, 32.2534) (105.9302, 32.1713) knots 0 0 0 1 1 1
  line L797 (105.9302, 32.1713) -> (105.9302, 31.5602)
  spline S740 degree 2 poles (105.9302, 31.5602) (105.7944, 31.6168) (105.4747, 31.6932) (105.3672, 31.6932) knots 0 0 0 1 2 2 2
  spline S741 degree 2 poles (105.3672, 31.6932) (105.2766, 31.6932) (105.1691, 31.6338) (105.1691, 31.58) knots 0 0 0 1 2 2 2
  spline S742 degree 2 poles (105.1691, 31.58) (105.1691, 31.5178) (105.2851, 31.4414) (105.4577, 31.3876) knots 0 0 0 1 2 2 2
  spline S743 degree 2 poles (105.4577, 31.3876) (105.7916, 31.2914) (106.083, 30.9859) (106.083, 30.7454) knots 0 0 0 1 2 2 2
  spline S744 degree 2 poles (108.2106, 30.0833) (108.1229, 30.0324) (107.7495, 29.9673) (107.5061, 29.9673) knots 0 0 0 1 2 2 2
  spline S745 degree 2 poles (107.5061, 29.9673) (107.161, 29.9673) (106.6177, 30.2474) (106.3207, 30.7482) (106.3207, 31.0622) knots 0 0 0 1 2 3 3 3
  spline S746 degree 2 poles (106.3207, 31.0622) (106.3207, 31.4357) (106.6375, 31.9705) (107.2232, 32.2534) (107.6108, 32.2534) knots 0 0 0 1 2 3 3 3
  spline S747 degree 2 poles (107.6108, 32.2534) (107.823, 32.2534) (108.1625, 32.1968) (108.2106, 32.1629) knots 0 0 0 1 2 2 2
  line L798 (108.2106, 32.1629) -> (108.2106, 31.4555)
  spline S748 degree 2 poles (108.2106, 31.4555) (108.1427, 31.5093) (107.8881, 31.5885) (107.7806, 31.5885) knots 0 0 0 1 2 2 2
  spline S749 degree 2 poles (107.7806, 31.5885) (107.5146, 31.5885) (107.2402, 31.3367) (107.2402, 31.1075) knots 0 0 0 1 2 2 2
  spline S750 degree 2 poles (107.2402, 31.1075) (107.2402, 30.8812) (107.509, 30.6322) (107.7466, 30.6322) knots 0 0 0 1 2 2 2
  spline S751 degree 2 poles (107.7466, 30.6322) (107.9984, 30.6322) (108.2106, 30.751) knots 0 0 0 1 1 1
  line L799 (108.2106, 30.751) -> (108.2106, 30.0833)
  spline S752 degree 2 poles (110.9947, 31.15) (110.9947, 30.5982) (110.3298, 29.9673) (109.7328, 29.9673) knots 0 0 0 1 2 2 2
  spline S753 degree 2 poles (109.7328, 29.9673) (109.1387, 29.9673) (108.4766, 30.5813) (108.4766, 31.1245) knots 0 0 0 1 2 2 2
  spline S754 degree 2 poles (108.4766, 31.1245) (108.4766, 31.4697) (108.7878, 31.9818) (109.3622, 32.2534) (109.7356, 32.2534) knots 0 0 0 1 2 3 3 3
  spline S755 degree 2 poles (109.7356, 32.2534) (110.1233, 32.2534) (110.692, 31.9676) (110.9947, 31.4612) (110.9947, 31.15) knots 0 0 0 1 2 3 3 3
  spline S756 degree 2 poles (110.0752, 31.1443) (110.0752, 31.5885) (109.7356, 31.5885) knots 0 0 0 1 1 1
  spline S757 degree 2 poles (109.7356, 31.5885) (109.3961, 31.5885) (109.3961, 31.1245) knots 0 0 0 1 1 1
  spline S758 degree 2 poles (109.3961, 31.1245) (109.3961, 30.6322) (109.7413, 30.6322) knots 0 0 0 1 1 1
  spline S759 degree 2 poles (109.7413, 30.6322) (110.0752, 30.6322) (110.0752, 31.1443) knots 0 0 0 1 1 1
  point P0 (0, 0)
  point P1 (0, 0)
  constraints: 4 other
extrude "Estrusione4" cut sketch "Schizzo4" against normal blind 1
